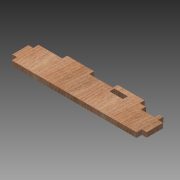
# Autodesk Inventor part: laterales
Saved by Autodesk Inventor 2015 (Build 190159000, 159)
## iProperties
Created: 2016-03-02
Part Number: laterales
Material: Wood (Birch)
Document SubType Name: Modeling
Designer: iberopuebla
Density: 0.55 g/cm^3
Appearance: Birch - Natural Polished
Author: iberopuebla
Autodesk Inventor part; units mm, degrees
ref_plane "YZ Plane" through (0, 0, 0) normal (1, 0, 0) x (0, 1, 0)
ref_plane "XZ Plane" through (0, 0, 0) normal (0, 1, 0) x (-1, 0, 0)
ref_plane "XY Plane" through (0, 0, 0) normal (0, 0, 1) x (1, 0, 0)
sketch "Sketch1" plane through (0, 0, 0) normal (0, 0, 1) x (1, 0, 0)
  line L0 (393.6245, -95.4118) -> (-70.3755, -95.4118)
  line L1 (17.6245, 22.5882) -> (117.6245, 22.5882)
  line L2 (117.6245, 22.5882) -> (117.6245, 4.5882)
  line L3 (17.6245, 4.5882) -> (17.6245, 22.5882)
  line L4 (-70.3755, 4.5882) -> (17.6245, 4.5882)
  line L5 (305.6245, 22.5882) -> (205.6245, 22.5882)
  line L6 (205.6245, 22.5882) -> (205.6245, 4.5882)
  line L7 (305.6245, 4.5882) -> (305.6245, 22.5882)
  line L8 (117.6245, 4.5882) -> (205.6245, 4.5882)
  line L9 (305.6245, 4.5882) -> (393.6245, 4.5882)
  line L10 (-88.3755, -15.4118) -> (-70.3755, -15.4118)
  line L11 (-70.3755, -75.4118) -> (-88.3755, -75.4118)
  line L12 (-88.3755, -75.4118) -> (-88.3755, -15.4118)
  line L13 (-70.3755, -95.4118) -> (-70.3755, -75.4118)
  line L14 (-70.3755, -15.4118) -> (-70.3755, 4.5882)
  line L15 (393.6245, -15.4118) -> (411.6245, -15.4118)
  line L16 (411.6245, -15.4118) -> (411.6245, -75.4118)
  line L17 (411.6245, -75.4118) -> (393.6245, -75.4118)
  line L18 (393.6245, 4.5882) -> (393.6245, -15.4118)
  line L19 (393.6245, -75.4118) -> (393.6245, -95.4118)
  point P0 (0, 0)
  dimension "d0" = 464
  dimension "d4" = 100
  dimension "d5" = 18
  dimension "d9" = 100
  dimension "d10" = 18
  dimension "d13" = 18
  dimension "d14" = 60
  dimension "d17" = 20
  dimension "d19" = 60
  dimension "d20" = 18
  dimension "d21" = 100
  dimension "d37" = 88
  dimension "d38" = 88
  dimension "d39" = 88
  constraints: 40 end point, 11 parallel, 9 perpendicular, 7 horizontal
  measures "d0" distance of L0.start L0.end
  measures "d4" distance of L2.end L3.start
  measures "d5" distance of L1.end L2.end
  measures "d9" distance of L7.start L6.end
  measures "d10" distance of L6.end L5.end
  measures "d13" distance of L11.start L11.end
  measures "d14" distance of L10.end L11.start
  measures "d17" distance between parallel lines of L0 L11
  measures "d19" distance between parallel lines of L17 L15
  measures "d20" distance of L15.start L15.end
  measures "d21" distance between parallel lines of L0 L9
  measures "d37" distance between parallel lines of L6 L2
  measures "d38" distance between parallel lines of L7 L18
  measures "d39" distance between parallel lines of L3 L14
extrude "Extrusion1" add sketch "Sketch1" along normal blind 18
sketch "Sketch2" plane through (0, 0, 18) normal (0, 0, 1) x (1, 0, 0)
  line L0 (-70.3755, -15.4118) -> (-71.5069, -14.2805)
  line L1 (-70.3755, -15.4118) -> (-68.7755, -15.4118) construction
  line L2 (-70.3755, -75.4118) -> (-71.5069, -76.5432)
  line L3 (17.6245, 4.5882) -> (16.4931, 5.7195)
  line L4 (17.6245, 4.5882) -> (19.2245, 4.5882) construction
  line L5 (117.6245, 4.5882) -> (118.7558, 5.7195)
  line L6 (205.6245, 4.5882) -> (204.4931, 5.7195)
  line L7 (305.6245, 4.5882) -> (306.7558, 5.7195)
  line L8 (393.6245, -15.4118) -> (394.7558, -14.2805)
  line L9 (393.6245, -75.4118) -> (394.7558, -76.5432)
  circle A0 centre (-71.5069, -14.2805) radius 1.6
  circle A1 centre (-71.5069, -76.5432) radius 1.6
  circle A2 centre (16.4931, 5.7195) radius 1.6
  circle A3 centre (118.7558, 5.7195) radius 1.6
  circle A4 centre (204.4931, 5.7195) radius 1.6
  circle A5 centre (306.7558, 5.7195) radius 1.6
  circle A6 centre (394.7558, -14.2805) radius 1.6
  circle A7 centre (394.7558, -76.5432) radius 1.6
  point P0 (0, 0)
  dimension "d22" = 1.6
  dimension "d23" = 135
  dimension "d24" = 1.6
  dimension "d25" = 135
  dimension "d26" = 3.2
  dimension "d27" = 3.2
  dimension "d28" = 3.2
  dimension "d29" = 3.2
  dimension "d30" = 3.2
  dimension "d32" = 3.2
  dimension "d33" = 3.2
  dimension "d34" = 3.2
  constraints: 20 end point, 8 centre point, 8 coincident, 6 perpendicular, 2 equal length, 2 horizontal, 1 parallel
  measures "d22" distance of L0.start L0.end
  measures "d23" angle of L1 L0
  measures "d24" distance of L3.start L3.end
  measures "d25" angle of L4 L3
  measures "d26" diameter of A0
  measures "d27" diameter of A1
  measures "d28" diameter of A2
  measures "d29" diameter of A3
  measures "d30" diameter of A4
  measures "d32" diameter of A5
  measures "d33" diameter of A6
  measures "d34" diameter of A7
extrude "Extrusion2" cut sketch "Sketch2" against normal blind 20
sketch "Sketch3" plane through (0, 0, 18) normal (0, 0, 1) x (1, 0, 0)
  line L0 (211.3165, 4.5882) -> (261.3165, 4.5882)
  line L1 (261.3165, 4.5882) -> (261.3165, -13.4118)
  line L2 (261.3165, -13.4118) -> (211.3165, -13.4118)
  line L3 (211.3165, -13.4118) -> (211.3165, 4.5882)
  line L4 (305.6245, 22.5882) -> (205.6245, 22.5882) projected
  line L5 (205.6245, 22.5882) -> (205.6245, 6.8509) projected
  line L6 (328.7435, 4.5882) -> (378.7435, 4.5882)
  line L7 (378.7435, 4.5882) -> (378.7435, -13.4118)
  line L8 (378.7435, -13.4118) -> (328.7435, -13.4118)
  line L9 (328.7435, -13.4118) -> (328.7435, 4.5882)
  line L10 (393.6245, 4.5882) -> (307.8872, 4.5882) projected
  point P0 (0, 0)
  dimension "d40" = 50
  dimension "d41" = 18
  dimension "d42" = 18
  dimension "d43" = 5.692
  dimension "d44" = 50
  dimension "d45" = 18
  dimension "d46" = 67.427
  dimension "d47" = 0
  constraints: 16 end point, 4 parallel, 2 horizontal, 2 perpendicular
  measures "d40" distance of L1.end L2.end
  measures "d41" distance of L0.end L1.end
  measures "d42" distance between parallel lines of L4 L0
  measures "d43" distance between parallel lines of L5 L3
  measures "d44" distance of L7.end L8.end
  measures "d45" distance of L6.end L7.end
  measures "d46" distance between parallel lines of L1 L9
  measures "d47" distance between parallel lines of L6 L10
extrude "Extrusion3" cut sketch "Sketch3" against normal blind 18
sketch "Sketch4" plane through (0, 0, 18) normal (0, 0, 1) x (1, 0, 0)
  line L0 (211.3165, 4.5882) -> (212.4478, 3.4568)
  line L1 (211.3165, 4.5882) -> (212.9165, 4.5882) construction
  line L2 (211.3165, -13.4118) -> (212.4478, -12.2805)
  line L3 (211.3165, -13.4118) -> (212.9165, -13.4118) construction
  line L4 (261.3165, -13.4118) -> (260.1851, -12.2805)
  line L5 (261.3165, 4.5882) -> (260.1851, 3.4568)
  circle A0 centre (212.4478, 3.4568) radius 1.6
  circle A1 centre (212.4478, -12.2805) radius 1.6
  circle A2 centre (260.1851, 3.4568) radius 1.6
  circle A3 centre (260.1851, -12.2805) radius 1.6
  line L6 (328.7435, -13.4118) -> (329.8748, -12.2805)
  line L7 (328.7435, -13.4118) -> (330.3435, -13.4118) construction
  line L8 (378.7435, -13.4118) -> (377.6121, -12.2805)
  circle A4 centre (377.6121, -12.2805) radius 1.6
  circle A5 centre (329.8748, -12.2805) radius 1.6
  point P0 (0, 0)
  dimension "d50" = 1.6
  dimension "d51" = 45
  dimension "d52" = 1.6
  dimension "d53" = 45
  dimension "d54" = 3.2
  dimension "d55" = 3.2
  dimension "d56" = 3.2
  dimension "d57" = 3.2
  dimension "d58" = 1.6
  dimension "d59" = 45
  dimension "d60" = 3.2
  dimension "d61" = 3.2
  constraints: 18 end point, 6 centre point, 6 coincident, 3 equal length, 3 horizontal, 3 perpendicular
  measures "d50" distance of L0.start L0.end
  measures "d51" angle of L0 L1
  measures "d52" distance of L2.start L2.end
  measures "d53" angle of L3 L2
  measures "d54" diameter of A0
  measures "d55" diameter of A1
  measures "d56" diameter of A2
  measures "d57" diameter of A3
  measures "d58" distance of L6.start L6.end
  measures "d59" angle of L7 L6
  measures "d60" diameter of A4
  measures "d61" diameter of A5
extrude "Extrusion4" cut sketch "Sketch4" against normal blind 20
body "Solid1"
